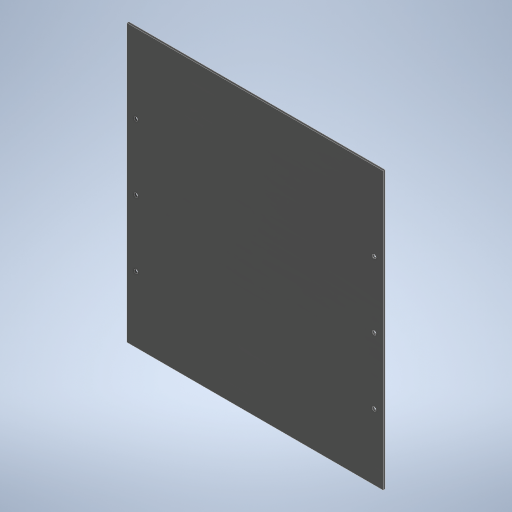
# Autodesk Inventor part: HCMUTE-CDT23-KXL_A05
Saved by Autodesk Inventor 2023 (Build 270158000, 158)
## iProperties
Created: 2023-11-20
Part Number: HCMUTE-CDT23-KXL_A05
Material: PMMA Plastic
Document SubType Name: Modeling
Designer: havie
Density: 1.188 g/cm^3
Appearance: Dark Gray
Author: havie
Autodesk Inventor part; units mm, degrees
ref_plane "YZ Plane" through (0, 0, 0) normal (1, 0, 0) x (0, 1, 0)
ref_plane "XZ Plane" through (0, 0, 0) normal (0, 1, 0) x (-1, 0, 0)
ref_plane "XY Plane" through (0, 0, 0) normal (0, 0, 1) x (1, 0, 0)
sketch "Sketch1" plane through (0, 0, 0) normal (0, 0, 1) x (1, 0, 0)
  line L0 (-200, 216) -> (200, 216)
  line L1 (200, 216) -> (200, -216)
  line L2 (200, -216) -> (-200, -216)
  line L3 (-200, -216) -> (-200, 216)
  line L4 (-200, 216) -> (200, -216) construction
  line L5 (200, 216) -> (-200, -216) construction
  point P0 (0, 0)
  dimension "d0" = 432
  dimension "d1" = 400
  constraints: 12 end point, 2 midpoint, 2 parallel, 1 horizontal, 1 perpendicular
  measures "d0" distance of L2.end L0.start
  measures "d1" distance of L1.end L2.end
extrude "Extrusion1" add sketch "Sketch1" along normal mid plane 3
sketch "Sketch2" plane through (0, 0, 1.5) normal (0, 0, 1) x (1, 0, 0)
  line L0 (-200, -216) -> (200, -216) projected
  line L1 (200, -216) -> (200, 216) projected
  point P0 (0, 0)
  point P1 (186, -113)
  point P2 (186, -10)
  point P3 (186, 93)
  dimension "d4" = 103
  dimension "d5" = 103
  dimension "d6" = 103
  dimension "d7" = 14
  constraints: 2 vertical alignment
  measures "d4" distance from line of L0 point (186, -113)
  measures "d5" distance of point (186, -10) point (186, -113)
  measures "d6" distance of point (186, 93) point (186, -10)
  measures "d7" distance from line of L1 point (186, -113)
hole "Hole1" at (186, -113, 1.5) at (186, -10, 1.5) at (186, 93, 1.5) direction (0, 0, -1) diameter 6 depth 14.2 tip angle 118
mirror "Mirror1" about plane through (0, 0, 0) normal (1, 0, 0) of "Hole1"
equation "\"d5\" = d4"
equation "\"d6\" = d5"
body "Solid1"
